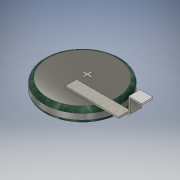
# Autodesk Inventor part: RJD2032C1ST1
Saved by Autodesk Inventor 2019.4 (Build 234330000, 330)
## iProperties
Created: 2020-05-13
Part Number: RJD2032C1ST1
Material: Generic
Document SubType Name: Modeling
Designer: Jorian Brusind
Density: 1 g/cm^3
Appearance: Default
Author: Jorian Brusind
Autodesk Inventor part; units mm, degrees
ref_plane "YZ Plane" through (0, 0, 0) normal (1, 0, 0) x (0, 1, 0)
ref_plane "XZ Plane" through (0, 0, 0) normal (0, 1, 0) x (-1, 0, 0)
ref_plane "XY Plane" through (0, 0, 0) normal (0, 0, 1) x (1, 0, 0)
sketch "Sketch1" plane through (0, 0, 0) normal (0, 1, 0) x (-1, 0, 0)
  circle A0 centre (0, 0) radius 10.01
  dimension "d0" = 20.02
  constraints: 1 centre point, 1 coincident
  measures "d0" diameter of A0
extrude "Extrusion1" add sketch "Sketch1" along normal blind 3.5
fillet "Fillet1" radius 1 1 edges at (10.01, 3.5, 0)
fillet "Fillet2" radius 1 1 edges at (10.01, 0, 0)
sketch "Sketch2" plane through (0, 3.5, 0) normal (0, 1, 0) x (1, 0, 0)
  line L0 (0, 0) -> (0, -1.5)
  line L1 (0, -1.5) -> (14, -1.5)
  line L2 (14, -1.5) -> (14, -4.5)
  line L3 (14, -4.5) -> (0, -4.5)
  line L4 (0, -4.5) -> (0, -1.5)
  dimension "d5" = 1.5
  dimension "d6" = 14
  dimension "d7" = 3
  constraints: 10 end point, 2 parallel, 1 horizontal, 1 perpendicular, 1 vertical
  measures "d5" distance of L0.start L0.end
  measures "d6" distance of L0.end L1.end
  measures "d7" distance of L1.end L2.end
extrude "Extrusion2" add sketch "Sketch2" along normal blind 0.4
sketch "Sketch3" plane through (0, 0, 0) normal (0, -1, 0) x (1, 0, 0)
  line L0 (0, 0) -> (0, -1.5)
  line L1 (0, -1.5) -> (11, -1.5)
  line L2 (11, -1.5) -> (11, -4.5)
  line L3 (11, -4.5) -> (0, -4.5)
  line L4 (0, -4.5) -> (0, -1.5)
  dimension "d10" = 1.5
  dimension "d11" = 11
  dimension "d12" = 3
  constraints: 10 end point, 2 parallel, 1 horizontal, 1 perpendicular, 1 vertical
  measures "d10" distance of L0.start L0.end
  measures "d11" distance of L0.end L1.end
  measures "d12" distance of L1.end L2.end
extrude "Extrusion3" add sketch "Sketch3" along normal blind 0.4
sketch "Sketch4" plane through (0, 0, 0) normal (0, 1, 0) x (1, 0, 0)
  line L0 (11, 4.5) -> (11, 1.5) projected
  line L1 (11, 1.5) -> (11, 4.5)
  line L2 (11, 4.5) -> (10.6, 4.5)
  line L3 (10.6, 4.5) -> (10.6, 1.5)
  line L4 (10.6, 1.5) -> (11, 1.5)
  point P0 (0, 0)
  dimension "d15" = 0.4
  constraints: 8 end point, 3 equal length, 1 perpendicular
  measures "d15" distance of L2.end L0.start
extrude "Extrusion4" add sketch "Sketch4" along normal blind 3.5
fillet "Fillet3" radius 0.4 1 edges at (11, -0.4, -3)
fillet "Fillet4" radius 0.4 1 edges at (10.6, 0, -3)
sketch "Sketch5" plane through (0, 3.5, 0) normal (0, 1, 0) x (1, 0, 0)
  line L0 (10.6, 4.5) -> (10.6, 1.5) projected
  line L1 (10.6, 1.5) -> (14, 1.5)
  line L2 (14, 1.5) -> (14, 4.5)
  line L3 (14, 4.5) -> (10.6, 4.5)
  line L4 (10.6, 4.5) -> (10.6, 1.5)
  point P0 (0, 0)
  dimension "d20" = 3
  dimension "d21" = 3.4
  constraints: 8 end point, 2 parallel, 1 horizontal, 1 perpendicular
  measures "d20" distance of L2.end L1.end
  measures "d21" distance of L0.end L1.end
extrude "Extrusion5" add sketch "Sketch5" along normal blind 0.4
sketch "Sketch6" plane through (0, 3.5, 0) normal (0, 1, 0) x (1, 0, 0)
  line L0 (-1.4984, 2.512) -> (1.5521, 2.512) construction
  line L1 (1.5521, 2.512) -> (1.5521, 0.1186) construction
  line L2 (1.5521, 0.1186) -> (-1.4984, 0.1186) construction
  line L3 (-1.4984, 0.1186) -> (-1.4984, 2.512) construction
  line L4 (1.231, 1.1511) -> (0.1985, 1.1511)
  line L5 (0.1985, 1.1511) -> (0.1985, 0.1186)
  line L6 (0.1985, 0.1186) -> (-0.1424, 0.1186)
  line L7 (-0.1424, 0.1186) -> (-0.1424, 1.1511)
  line L8 (-0.1424, 1.1511) -> (-1.1748, 1.1511)
  line L9 (-1.1748, 1.1511) -> (-1.1748, 1.4796)
  line L10 (-1.1748, 1.4796) -> (-0.1424, 1.4796)
  line L11 (-0.1424, 1.4796) -> (-0.1424, 2.512)
  line L12 (-0.1424, 2.512) -> (0.1985, 2.512)
  line L13 (0.1985, 2.512) -> (0.1985, 1.4796)
  line L14 (0.1985, 1.4796) -> (1.231, 1.4796)
  line L15 (1.231, 1.4796) -> (1.231, 1.1511)
  point P0 (0, 0)
  constraints: 2 other
extrude "Extrusion6" add sketch "Sketch6" along normal mid plane 0.4
body "Solid1"
